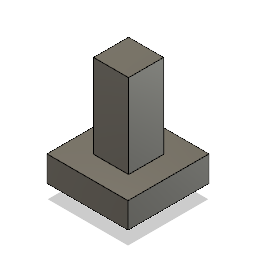
revB-switch-design (Autodesk Fusion 360 design; units mm, degrees)
Autodesk Fusion 360 part; units mm, degrees
sketch "Sketch1" plane through (0, 0, 0) normal (0, 1, 0) x (1, 0, 0)
  line L0 (0, 0) -> (6, 0)
  line L1 (6, 0) -> (6, -6)
  line L2 (6, -6) -> (0, -6)
  line L3 (0, -6) -> (0, 0)
  dimension "d1" = 6
  dimension "d2" = 6
  measures "d1" distance of L0.start L0.end
  measures "d2" distance of L0.end L1.end
extrude "Extrude1" add sketch "Sketch1" along normal blind 1.9
sketch "Sketch2" plane through (0, 1.9, 0) normal (0, 1, 0) x (-1, 0, 0)
  line L0 (0, 6) -> (-6, 6)
  line L1 (-6, 6) -> (-6, 0)
  line L2 (-6, 0) -> (0, 0)
  line L3 (0, 0) -> (0, 6)
  line L4 (-1.7485, 1.7053) -> (-4.3485, 1.7053)
  line L5 (-4.3485, 1.7053) -> (-4.3485, 4.3053)
  line L6 (-4.3485, 4.3053) -> (-1.7485, 4.3053)
  line L7 (-1.7485, 4.3053) -> (-1.7485, 1.7053)
  dimension "d5" = 2.6
  dimension "d6" = 2.6
  measures "d5" distance of L4.start L6.end
  measures "d6" distance of L4.start L4.end
extrude "Extrude2" add sketch "Sketch2" along normal blind 6.2 contours L4 L5 L6 L7
sketch "Sketch3" plane through (0, 0, 0) normal (0, -1, 0) x (1, 0, 0)
  line L0 (6, 6) -> (0, 6)
  line L1 (0, 6) -> (0, 0)
  line L2 (0, 0) -> (6, 0)
  line L3 (6, 0) -> (6, 6)
  line L4 (1.7485, 4.3053) -> (4.3485, 4.3053)
  line L5 (4.3485, 4.3053) -> (4.3485, 1.7053)
  line L6 (4.3485, 1.7053) -> (1.7485, 1.7053)
  line L7 (1.7485, 1.7053) -> (1.7485, 4.3053)
  point P0 (1.7485, 4.3053)
  point P1 (4.3485, 1.7053)
extrude "Extrude3" add sketch "Sketch3" along normal blind 1 contours L4 L5 L6 L7
